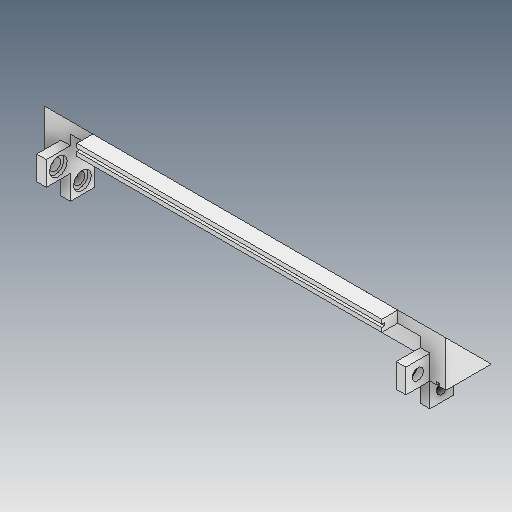
# Autodesk Inventor part: angles_struts
Saved by Autodesk Inventor 2027 (Build 310192060, 192F)
## iProperties
Created: 2026-07-26
Part Number: angles_struts
Material: ABS Plastic
Document SubType Name: Modeling
Designer: prest
Density: 1.06 g/cm^3
Appearance: Smooth - White
Author: prest
Autodesk Inventor part; units mm, degrees
ref_plane "YZ Plane" through (0, 0, 0) normal (1, 0, 0) x (0, 1, 0)
ref_plane "Work Plane1" through (0, 0, 0) normal (0, 0.7071068, -0.7071068) x (-1, 0, 0)
sketch "Sketch2" plane through (0, 0, 0) normal (0, 0.7071068, -0.7071068) x (-1, 0, 0)
  line L0 (-125, 15) -> (125, 15)
  line L1 (125, 15) -> (125, -15)
  line L2 (125, -15) -> (-125, -15)
  line L3 (-125, -15) -> (-125, 15)
  point P0 (0, 0)
  point P1 (-125, 0)
  point P2 (0, -15)
  dimension "d6" = 250
  dimension "d13" = 30
  constraints: 8 end point, 2 midpoint, 2 parallel, 1 horizontal, 1 horizontal alignment, 1 perpendicular, 1 vertical alignment
  measures "d6" distance of L0.start L0.end
  measures "d13" distance of L2.end L0.start
extrude "Extrusion2" add sketch "Sketch2" along normal blind 5
ref_plane "Work Plane2" through (-115, -10.6066, -10.6066) normal (-1, 0, 0) x (0, -0.7071068, 0.7071068)
sketch "Sketch7" plane through (-115, -10.6066, -10.6066) normal (-1, 0, 0) x (0, -0.7071068, 0.7071068)
  line L0 (0, 30) -> (4.3934, 25.6066)
  line L1 (4.3934, 4.3934) -> (0, 0)
  line L2 (15, 15) -> (25.6066, 25.6066)
  line L3 (25.6066, 25.6066) -> (15, 36.2132)
  line L4 (15, 36.2132) -> (4.3934, 25.6066)
  line L5 (15, 15) -> (25.6066, 4.3934)
  line L6 (25.6066, 4.3934) -> (15, -6.2132)
  line L7 (15, -6.2132) -> (4.3934, 4.3934)
  line L8 (0, 0) -> (0, 30) projected
  point P0 (0, -9.4286)
  dimension "d21" = 15
  dimension "d22" = 15
  dimension "d23" = 45
  dimension "d24" = 45
  constraints: 16 end point, 8 perpendicular, 2 coincident, 1 collinear
  measures "d21" distance of L3.end L0.end
  measures "d22" distance of L2.end L3.end
  measures "d23" angle of L8 L0
  measures "d24" angle of L8 L1
extrude "Extrusion6" add sketch "Sketch7" against normal blind 6
sketch "Sketch8" plane through (-125, -10.6066, -10.6066) normal (-1, 0, 0) x (0, -0.7071068, 0.7071068)
  line L0 (0, 0) -> (-5, -5)
  line L1 (-5, -5) -> (-5, 0)
  line L2 (0, 0) -> (-5, 0) projected
  line L3 (0, 30) -> (4.3934, 25.6066) projected
  line L4 (0, 30) -> (-5, 35)
  line L5 (0, 30) -> (-5, 30) projected
  line L6 (-5, 35) -> (-5, 30)
  point P0 (0, 15)
  constraints: 8 end point, 2 perpendicular, 1 collinear, 1 vertical
extrude "Extrusion7" add sketch "Sketch8" against normal up to surface (250 mm away) from surface at 0
sketch "Sketch9" plane through (-109, -10.6066, -10.6066) normal (1, 0, 0) x (0, -0.7071068, -0.7071068)
  line L0 (6.2132, -15) -> (-4.3934, -4.3934) projected
  line L1 (-36.2132, -15) -> (-25.6066, -25.6066) projected
  line L2 (6.2132, -15) -> (-36.2132, -15) construction
  line L3 (-30, 0) -> (-25.6066, -4.3934) projected
  line L4 (-25.6066, -25.6066) -> (-25.6066, -4.3934) construction
  line L5 (-4.3934, -25.6066) -> (-4.3934, -4.3934) construction
  point P0 (-15, 0)
  point P1 (-4.3934, -15)
  point P2 (-25.6066, -15)
  constraints: 6 end point, 2 vertical, 1 horizontal, 1 midpoint, 1 point on line
hole "Hole1" at (-109, -18.1066, 3.1066) at (-109, -3.1066, 18.1066) direction (-1, 0, 0) diameter 7 end through all counterbore diameter 11 counterbore depth 2
sketch "Sketch11" plane through (-115, -10.6066, -10.6066) normal (-1, 0, 0) x (0, 0.7071068, 0.7071068)
  line L0 (4.3934, -4.3934) -> (0, 0) projected
  line L1 (15, -15) -> (0, 0)
  line L2 (0, 0) -> (30, 0) projected
  line L3 (25.6066, -25.6066) -> (15, -15) projected
  line L4 (15, -15) -> (30, 0)
  point P0 (15, 0)
  constraints: 4 end point, 1 collinear, 1 perpendicular
extrude "Extrusion9" add sketch "Sketch11" along normal blind 10
mirror "Mirror6" about plane through (0, 0, 0) normal (1, 0, 0) of "Hole1", "Extrusion6"
sketch "Sketch12" plane through (115, -10.6066, 25.6066) normal (1, 0, 0) x (0, 0, -1)
  line L0 (15, 21.2132) -> (36.2132, 0) projected
  line L1 (0, 0) -> (15, 0) projected
  line L2 (36.2132, 0) -> (15, 0)
  line L3 (15, 0) -> (15, 21.2132)
  point P0 (25.6066, 10.6066)
  constraints: 4 end point, 1 collinear, 1 perpendicular
extrude "Extrusion10" add sketch "Sketch12" along normal blind 10
sketch "Sketch13" plane through (-125, -10.6066, -17.6777) normal (0, -1, 0) x (1, 0, 0)
  line L0 (250, 0) -> (0, 0) projected
  line L1 (234, 7.0711) -> (16, 7.0711) projected
  line L2 (220, 0) -> (30, 0)
  line L3 (30, 0) -> (30, 7.0711)
  line L4 (30, 7.0711) -> (220, 7.0711)
  line L5 (220, 7.0711) -> (220, 0)
  line L6 (250, 28.2843) -> (250, 0) projected
  line L7 (0, 28.2843) -> (0, 0) projected
  point P0 (125, 17.6777)
  point P1 (220, 3.5355)
  point P2 (220, 7.0711)
  point P3 (30, 0)
  dimension "d42" = 30
  dimension "d43" = 30
  constraints: 8 end point, 2 parallel, 2 point on line, 1 horizontal, 1 midpoint, 1 perpendicular
  measures "d42" distance from line of point (220, 3.536) L6
  measures "d43" distance between parallel lines of L7 L3
extrude "Extrusion11" add sketch "Sketch13" along normal blind 10
sketch "Sketch14" plane through (-125, 17.6777, 10.6066) normal (0, 0, 1) x (1, 0, 0)
  line L0 (250, 0) -> (0, 0) projected
  line L1 (16, -7.0711) -> (234, -7.0711) projected
  line L2 (30, 0) -> (220, 0)
  line L3 (220, 0) -> (220, -7.0711)
  line L4 (220, -7.0711) -> (30, -7.0711)
  line L5 (30, -7.0711) -> (30, 0)
  line L6 (0, 0) -> (0, -28.2843) projected
  line L7 (250, -28.2843) -> (250, 0) projected
  line L8 (30, 0) -> (220, 0)
  line L9 (220, 0) -> (220, -7.0711)
  line L10 (220, -7.0711) -> (30, -7.0711)
  line L11 (30, -7.0711) -> (30, 0)
  point P0 (125, -17.6777)
  point P1 (30, -7.0711)
  dimension "d46" = 30
  dimension "d47" = 30
  constraints: 16 end point, 4 parallel, 2 horizontal, 2 perpendicular, 2 point on line
  measures "d46" distance between parallel lines of L6 L5
  measures "d47" distance between parallel lines of L3 L7
extrude "Extrusion12" add sketch "Sketch14" along normal blind 10
sketch "Sketch15" plane through (-125, -10.6066, 10.6066) normal (0, 0, 1) x (1, 0, 0)
  line L0 (30, 0) -> (0, 0) projected
  line L1 (4.1, 0) -> (5.9, 0)
  line L2 (5.9, 0) -> (5.9, 1.8)
  line L3 (5.9, 1.8) -> (4.1, 1.8)
  line L4 (4.1, 1.8) -> (4.1, 0)
  line L5 (0, 28.2843) -> (0, 0) projected
  point P0 (125, 10.6066)
  point P1 (5.9, 0)
  dimension "d50" = 1.8
  dimension "d51" = 1.8
  dimension "d52" = 4.1
  constraints: 8 end point, 2 parallel, 1 horizontal, 1 perpendicular, 1 point on line
  measures "d50" distance of L1.end L2.end
  measures "d51" distance of L2.end L3.end
  measures "d52" distance between parallel lines of L4 L5
extrude "Extrusion13" cut sketch "Sketch15" against normal blind 1.8
mirror "Mirror7" about plane through (0, 0, 0) normal (1, 0, 0) of "Extrusion13"
sketch "Sketch16" plane through (-125, 17.6777, 20.6066) normal (0, 0, 1) x (1, 0, 0)
  line L0 (30, 0) -> (30, -7.0711) projected
  line L1 (30, -3.5355) -> (220, -3.5355)
  line L2 (220, -7.0711) -> (220, 0) projected
  line L3 (30, -2.6355) -> (220, -2.6355)
  line L4 (30, -4.4355) -> (220, -4.4355)
  line L5 (220, -4.4355) -> (220, -2.6355)
  line L6 (30, -4.4355) -> (30, -2.6355)
  line L7 (30, -7.0711) -> (220, -7.0711) projected
  point P0 (125, -17.6777)
  point P1 (30, -4.4355)
  dimension "d55" = 1.8
  constraints: 10 end point, 2 midpoint, 2 point on line, 2 symmetric about line, 1 collinear, 1 horizontal, 1 perpendicular
  measures "d55" diameter of L3 L1
extrude "Extrusion14" cut sketch "Sketch16" against normal blind 1.8 contours L3 L2 L1 L0 | L1 L2 L4 L0
sketch "Sketch17" plane through (-125, -20.6066, -17.6777) normal (0, -1, 0) x (1, 0, 0)
  line L0 (30, 0) -> (30, 7.0711) projected
  line L1 (30, 3.5355) -> (220, 3.5355)
  line L2 (220, 7.0711) -> (220, 0) projected
  line L3 (30, 2.6355) -> (220, 2.6355)
  line L4 (30, 4.4355) -> (220, 4.4355)
  line L5 (30, 4.4355) -> (30, 2.6355)
  line L6 (220, 4.4355) -> (220, 2.6355)
  point P0 (125, 17.6777)
  point P1 (30, 4.4355)
  dimension "d58" = 1.8
  constraints: 10 end point, 2 midpoint, 2 point on line, 2 symmetric about line, 2 vertical, 1 perpendicular
  measures "d58" diameter of L3 L1
extrude "Extrusion15" cut sketch "Sketch17" against normal blind 1.8
equation "\"d43\" = d42"
body "Solid2"
